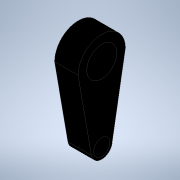
# Autodesk Inventor part: SLIDER CRANK-FIRST REVOLUTER
Saved by Autodesk Inventor 2021 (Build 250183000, 183)
## iProperties
Created: 2021-07-25
Part Number: SLIDER CRANK-FIRST REVOLUTER
Material: Generic
Document SubType Name: Modeling
Designer: HP
Density: 1 g/cm^3
Appearance: Default
Author: HP
Autodesk Inventor part; units mm, degrees
ref_plane "YZ Plane" through (0, 0, 0) normal (1, 0, 0) x (0, 1, 0)
ref_plane "XZ Plane" through (0, 0, 0) normal (0, 1, 0) x (-1, 0, 0)
ref_plane "XY Plane" through (0, 0, 0) normal (0, 0, 1) x (1, 0, 0)
sketch "Sketch1" plane through (0, 0, 0) normal (1, 0, 0) x (0, 1, 0)
  circle A0 centre (10.7653, 0) radius 3.556
  circle A1 centre (10.7653, 0) radius 2.2479
  circle A2 centre (-0.3599, 0) radius 1.5875
  line L0 (10.7653, -3.556) -> (-0.3599, -1.5875)
  line L1 (-0.6332, 1.5638) -> (10.7653, 3.556)
  circle A3 centre (-0.3599, 0) radius 1.2276
  point P0 (0, 0)
  dimension "d0" = 7.112
  dimension "d1" = 4.4958
  dimension "d3" = 3.175
  constraints: 4 centre point, 4 end point, 4 point on circle, 2 coincident, 1 tangent
  measures "d0" diameter of A0
  measures "d1" diameter of A1
  measures "d3" diameter of A2
extrude "Extrusion1" add sketch "Sketch1" along normal blind 3.5306 contours A0 L0 L1 | A0 L0 A2 L1 | A2
body "Solid1"
